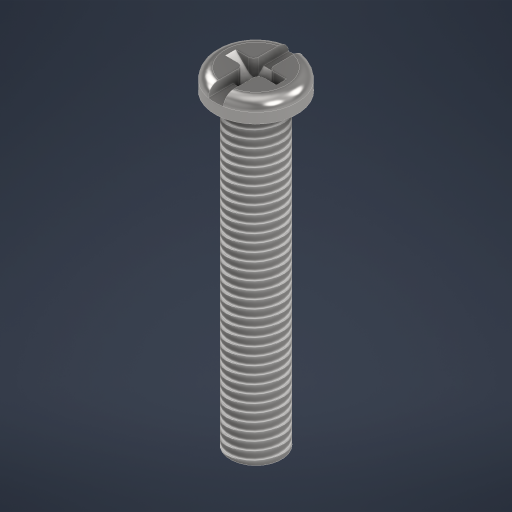
# Autodesk Inventor part: Langbektang houder
Saved by Autodesk Inventor 2023.2 (Build 272271000, 271)
## iProperties
Created: 2020-09-09
Part Number: Langbektang houder
Material: Steel, Mild
Document SubType Name: Modeling
Designer: nathan.bollaert
Density: 7.85 g/cm^3
Appearance: Semi-Polished
Author: nathan.bollaert
Autodesk Inventor part; units mm, degrees
ref_plane "YZ Plane" through (0, 0, 0) normal (1, 0, 0) x (0, 1, 0)
ref_plane "XZ Plane" through (0, 0, 0) normal (0, 1, 0) x (-1, 0, 0)
ref_plane "XY Plane" through (0, 0, 0) normal (0, 0, 1) x (1, 0, 0)
sketch "Sketch1" plane through (0, 0, 0) normal (0, 1, 0) x (-1, 0, 0)
  circle A0 centre (0, 0) radius 2.5
  circle A1 centre (0, 0) radius 4
  dimension "d228" = 5
  dimension "d229" = 8
  constraints: 2 centre point, 2 coincident
  measures "d228" diameter of A0
  measures "d229" diameter of A1
extrude "Extrusion1" add sketch "Sketch1" against normal blind 30 contours A0
extrude "Extrusion2" add sketch "Sketch1" along normal blind 2 contours A0 | A1
fillet "Fillet1" radius 0.5 1 edges at (4, 2, 0)
sketch "Sketch2" plane through (0, 2, 0) normal (0, 1, 0) x (1, 0, 0)
  line L0 (0.75, -4) -> (-0.75, -4)
  line L1 (-0.75, -4) -> (-0.75, 4)
  line L2 (-0.75, 4) -> (0.75, 4)
  line L3 (0.75, 4) -> (0.75, -4)
  circle A0 centre (0, 0) radius 4 projected
  line L4 (0, -4) -> (0, 4)
  line L5 (-2.5, -0.5) -> (2.5, -0.5)
  line L6 (2.5, -0.5) -> (2.5, 0.5)
  line L7 (2.5, 0.5) -> (-2.5, 0.5)
  line L8 (-2.5, 0.5) -> (-2.5, -0.5)
  line L9 (-4, 0) -> (4, 0)
  line L10 (-0.75, -2.5) -> (0.75, -2.5)
  line L11 (0.75, -2.5) -> (0.75, 2.5)
  line L12 (0.75, 2.5) -> (-0.75, 2.5)
  line L13 (-0.75, 2.5) -> (-0.75, -2.5)
  line L14 (-0.5, 0.5) -> (0.5, 0.5)
  line L15 (0.5, 0.5) -> (0.5, -0.5)
  line L16 (0.5, -0.5) -> (-0.5, -0.5)
  line L17 (-0.5, -0.5) -> (-0.5, 0.5)
  point P0 (-0.75, -3.9291)
  point P1 (0.75, -3.9291)
  point P2 (0.75, 3.9291)
  point P3 (-0.75, 3.9291)
  point P4 (0.75, 0.5)
  point P5 (-0.75, 0.5)
  point P6 (-0.75, -0.5)
  point P7 (0.75, -0.5)
  dimension "d234" = 8
  dimension "d235" = 1.5
  dimension "d236" = 1
  dimension "d237" = 5
  dimension "d238" = 5
  dimension "d243" = 1
  dimension "d244" = 1
  constraints: 36 end point, 8 parallel, 5 horizontal, 4 perpendicular, 4 point on circle, 2 midpoint, 2 point on line, 1 coincident, 1 vertical, 6 other
  measures "d234" distance of L0.end L1.end
  measures "d235" distance of L1.end L2.end
  measures "d236" distance of L7.end L5.start
  measures "d237" distance of L5.start L5.end
  measures "d238" distance of L12.end L10.start
  measures "d243" distance of L16.end L14.start
  measures "d244" distance between parallel lines of L15 L17
extrude "Extrusion3" cut sketch "Sketch2" against normal blind 2 contours L5 L17 L9 L4 | L4 L9 L15 L5 | L9 L17 L7 L4 | L4 L7 L15 L9
chamfer "Chamfer1" distance 2 angle 45 4 edges at (-0.5, 2, 0) (0.5, 2, 0) (0, 2, 0.5) (0, 2, -0.5)
extrude "Extrusion4" cut sketch "Sketch2" against normal blind 1 contours L4 L10 L3 A0 | A0 L1 L10 L4 | L10 L1 L5 L4 | L4 L5 L3 L10 | L3 L12 L4 A0 | A0 L4 L12 L1 | L3 L7 L4 L12 | L12 L4 L7 L1
extrude "Extrusion5" add sketch "Sketch2" against normal blind 2 contours L3 L5 L6 L9 A0 | A0 L9 L8 L5 L1 | L9 L6 L7 L3 A0 | A0 L1 L7 L8 L9
thread "Thread1" size "M5x0.8" class "6g" standard "ANSI Metric M Profile" full length
fillet "Fillet2" radius 1 2 edges at (4, 2, 0) (-4, 2, 0)
fillet "Fillet3" radius 0.5 4 edges at (-0.75, 1.125, -0.5) (0.75, 1.125, -0.5) (-0.75, 1.125, 0.5) (0.75, 1.125, 0.5)
body "Solid5"
